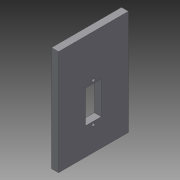
# Autodesk Inventor part: gripper_servo
Saved by Autodesk Inventor 2014 (Build 180170000, 170)
## iProperties
Created: 2014-04-25
Part Number: gripper_servo
Material: Generic
Document SubType Name: Modeling
Designer: t_emanb
Density: 1 g/cm^3
Appearance: Default
Author: t_emanb
Autodesk Inventor part; units mm, degrees
ref_plane "YZ Plane" through (0, 0, 0) normal (1, 0, 0) x (0, 1, 0)
ref_plane "XZ Plane" through (0, 0, 0) normal (0, 1, 0) x (-1, 0, 0)
ref_plane "XY Plane" through (0, 0, 0) normal (0, 0, 1) x (1, 0, 0)
sketch "Sketch1" plane through (0, 0, 0) normal (1, 0, 0) x (0, 1, 0)
  line L0 (0, 0) -> (76.2, 0)
  line L1 (76.2, 0) -> (76.2, 50.8)
  line L2 (76.2, 50.8) -> (0, 50.8)
  line L3 (0, 50.8) -> (0, 0)
  line L4 (0, 25.4) -> (76.2, 25.4) construction
  circle A0 centre (25.4, 25.4) radius 3.81
  line L5 (43.5104, 25.4) -> (19.7104, 25.4) construction
  line L6 (19.7104, 19.7) -> (19.7104, 31.1)
  line L7 (19.7104, 31.1) -> (43.5104, 31.1)
  line L8 (43.5104, 31.1) -> (43.5104, 19.7)
  line L9 (43.5104, 19.7) -> (19.7104, 19.7)
  line L10 (31.6104, 19.7) -> (31.6104, 31.1) construction
  circle A1 centre (17.6022, 25.4) radius 1
  circle A2 centre (45.6186, 25.4) radius 1
  line L11 (25.4, 19.7) -> (25.4, 31.1) construction
  dimension "d0" = 76.2
  dimension "d1" = 50.8
  dimension "d2" = 23.8
  dimension "d3" = 11.4
  dimension "d4" = 2
  dimension "d5" = 2.1082
  dimension "d6" = 5.6896
  dimension "d7" = 25.4
  constraints: 24 end point, 7 midpoint, 4 parallel, 3 centre point, 3 point on line, 2 perpendicular, 1 collinear, 1 horizontal, 1 symmetric about line, 1 other
  measures "d0" distance of L0.start L0.end
  measures "d1" distance of L2.end L0.start
  measures "d2" distance of L5.start L5.end
  measures "d3" distance of L6.start L7.start
  measures "d4" diameter of A1
  measures "d5" distance from line of A1.centre L6
  measures "d6" distance between parallel lines of L6 L11
  measures "d7" distance between parallel lines of L3 L11
extrude "Extrusion1" add sketch "Sketch1" along normal blind 5.08 contours L3 L2 L1 L0
body "Solid1"
